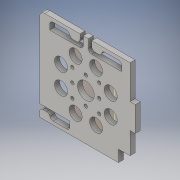
# Autodesk Inventor part: SideRotated
Saved by Autodesk Inventor 2016 SP1 (Build 200210100, 210)
## iProperties
Created: 2015-06-30
Part Number: SideRotated
Material: Generic
Document SubType Name: Modeling
Designer: Rodrigo
Density: 1 g/cm^3
Appearance: Default
Author: Rodrigo
Autodesk Inventor part; units mm, degrees
ref_plane "YZ Plane" through (0, 0, 0) normal (1, 0, 0) x (0, 1, 0)
ref_plane "XZ Plane" through (0, 0, 0) normal (0, 1, 0) x (-1, 0, 0)
ref_plane "XY Plane" through (0, 0, 0) normal (0, 0, 1) x (1, 0, 0)
ref_plane "Work Plane1" through (0, 0, 0) normal (0, 0, 1) x (1, 0, 0)
sketch "Sketch1" plane through (0, 0, 0) normal (0, 0, 1) x (1, 0, 0)
  circle A0 centre (6.5, 20.75) radius 1
  circle A1 centre (6.5, 4.75) radius 1
  circle A2 centre (22.5, 20.75) radius 1
  circle A3 centre (22.5, 4.75) radius 1
  line L0 (-13, -14.75) -> (43.896, -14.75)
  line L1 (43.896, -14.75) -> (43.896, 40.25)
  line L2 (43.896, 40.25) -> (-13, 40.25)
  line L3 (-13, 40.25) -> (-13, -14.75)
  circle A4 centre (22.5, 12.75) radius 1 projected
  circle A5 centre (14.5, 20.75) radius 1 projected
  circle A6 centre (14.5, 4.75) radius 1 projected
  circle A7 centre (6.5, 12.75) radius 1 projected
  point P0 (0, 0)
  point P1 (14.5, 12.75)
  dimension "d1" = 55
  dimension "d102" = 29.396
  dimension "d103" = 27.5
  dimension "d107" = 2
  dimension "d108" = 2
  dimension "d109" = 2
  dimension "d110" = 2
  constraints: 8 end point, 4 centre point, 2 parallel, 1 horizontal, 1 perpendicular
  measures "d1" distance of L1.end L0.end
  measures "d102" distance from line of L1 point (14.5, 12.75)
  measures "d103" distance from line of L3 point (14.5, 12.75)
  measures "d107" diameter of A0
  measures "d108" diameter of A2
  measures "d109" diameter of A3
  measures "d110" diameter of A1
extrude "Extrusion3" add sketch "Sketch1" along normal blind 3
sketch "Sketch4" plane through (0, 0, 3) normal (0, 0, 1) x (1, 0, 0)
  line L0 (42, 40.25) -> (-13, 40.25) construction
  line L1 (14.5, 40.25) -> (14.5, 12.75) construction
  line L2 (-13, 12.75) -> (14.5, 12.75) construction
  line L3 (42, 40.25) -> (-13, 40.25)
  line L4 (5, 38.2532) -> (-7, 38.25)
  line L5 (13, 40.25) -> (-7, 40.25)
  line L6 (-7, 38.25) -> (-7, 33.25)
  line L7 (-7, 33.25) -> (13, 33.25)
  line L8 (13, 40.25) -> (13, 33.25)
  line L9 (5, -7.75) -> (-13, -7.75)
  circle A0 centre (14.5, 12.75) radius 5
  line L10 (14.5, 12.75) -> (20.6229, 27.5321)
  line L11 (14.5, 12.75) -> (30.5, 12.75) construction
  circle A1 centre (20.6229, 27.5321) radius 3.895
  circle A2 centre (8.3771, 27.5321) radius 3.895
  circle A3 centre (-0.2821, 18.8729) radius 3.895
  circle A4 centre (-0.2821, 6.6271) radius 3.895
  circle A5 centre (8.3771, -2.0321) radius 3.895
  circle A6 centre (20.6229, -2.0321) radius 3.895
  circle A7 centre (29.2821, 6.6271) radius 3.895
  circle A8 centre (29.2821, 18.8729) radius 3.895
  line L12 (5, -12.75) -> (5, -7.75)
  line L13 (5, -12.75) -> (-7, -12.75)
  line L14 (-13, -7.75) -> (-13, -9.75)
  line L15 (-13, 40.25) -> (-13, -14.75) projected
  line L16 (-13, -9.75) -> (-7, -9.75)
  line L17 (-7, -9.75) -> (-7, -12.75)
  line L18 (-13, -14.75) -> (43.896, -14.75) projected
  line L19 (5, 38.2532) -> (5, 35.25)
  line L20 (5, 35.25) -> (11, 35.25)
  line L21 (11, 35.25) -> (11, 40.25)
  line L22 (24, 38.2532) -> (36, 38.25)
  line L23 (16, 40.25) -> (36, 40.25)
  line L24 (36, 38.25) -> (36, 33.25)
  line L25 (36, 33.25) -> (16, 33.25)
  line L26 (16, 40.25) -> (16, 33.25)
  line L27 (24, 38.2532) -> (24, 35.25)
  line L28 (24, 35.25) -> (18, 35.25)
  line L29 (18, 35.25) -> (18, 40.25)
  point P0 (0, 0)
  dimension "d66" = 20
  dimension "d105" = 10
  dimension "d111" = 16
  dimension "d112" = 67.5
  dimension "d113" = 7.79
  dimension "d116" = 360
  dimension "d119" = 12
  dimension "d120" = 2
  dimension "d121" = 5
  dimension "d122" = 2
  dimension "d123" = 18
  dimension "d124" = 2
  dimension "d125" = 5
  dimension "d126" = 2
  dimension "d127" = 2
  dimension "d128" = 6
  dimension "d129" = 12
  dimension "d130" = 6
  constraints: 56 end point, 9 centre point, 9 symmetric about line, 5 point on line, 4 horizontal, 4 perpendicular, 4 vertical, 2 coincident, 1 collinear, 1 equal length, 1 midpoint, 17 other
  measures "d66" distance of L5.start L5.end
  measures "d105" diameter of A0
  measures "d111" distance of L10.start L10.end
  measures "d112" angle of L11 L10
  measures "d113" diameter of A1
  measures "d119" distance of L12.start L13.end
  measures "d120" distance of L9.end L14.end
  measures "d121" distance between parallel lines of L18 L16
  measures "d122" distance between parallel lines of L18 L13
  measures "d123" distance of L9.start L9.end
  measures "d124" distance of L5.end L4.end
  measures "d125" distance of L20.end L21.end
  measures "d126" distance between parallel lines of L20 L7
  measures "d127" distance between parallel lines of L8 L21
  measures "d128" distance between parallel lines of L15 L6
  measures "d129" distance of L4.start L4.end
  measures "d130" distance of L19.end L20.end
extrude "Extrusion2" cut sketch "Sketch4" against normal through all
fillet "Fillet3" radius 2 14 edges at (-7, 38.25, 1.5) (5, 38.2532, 1.5) (13, 33.25, 1.5) (5, -12.75, 1.5) (-7, -12.75, 1.5) (-7, -9.75, 1.5) (-13, -9.75, 1.5) (5, 35.25, 1.5) (11, 35.25, 1.5) (16, 33.25, 1.5) (24, 35.25, 1.5) (18, 35.25, 1.5) (36, 38.25, 1.5) (24, 38.2532, 1.5)
sketch "Sketch6" plane through (0, 0, 3) normal (0, 0, 1) x (1, 0, 0)
  line L0 (43.896, 40.25) -> (-13, 40.25) projected
  line L1 (43.896, 40.25) -> (40.796, 40.25)
  line L2 (40.796, 40.25) -> (40.796, 20.2)
  line L3 (40.796, 20.2) -> (43.896, 20.2)
  line L4 (43.896, 20.2) -> (43.896, 40.25)
  line L5 (43.896, -14.75) -> (43.896, 40.25) construction
  line L6 (43.896, 12.75) -> (-13, 12.75) construction
  line L7 (-13, 40.25) -> (-13, -14.75) construction
  line L8 (43.896, -14.75) -> (40.796, -14.75)
  line L9 (40.796, -7.75) -> (40.796, 5.3)
  line L10 (40.796, 5.3) -> (43.896, 5.3)
  line L11 (43.896, 5.3) -> (43.896, -14.75)
  line L12 (43.896, -14.75) -> (33.896, -14.75)
  line L13 (33.896, -14.75) -> (33.896, -7.75)
  line L14 (33.896, -7.75) -> (40.796, -7.75)
  line L15 (43.896, -7.75) -> (43.896, -14.75)
  point P0 (0, 0)
  point P1 (36.3284, 40.25)
  point P2 (-13, -7.75)
  dimension "d96" = 3.1
  dimension "d97" = 20.05
  dimension "d100" = 10
  dimension "d101" = 7
  constraints: 26 end point, 4 parallel, 3 horizontal, 3 symmetric about line, 2 midpoint, 2 perpendicular
  measures "d96" distance of L3.end L2.end
  measures "d97" distance of L2.end L1.end
  measures "d100" distance of L13.end L15.start
  measures "d101" distance of L12.end L13.end
extrude "Extrusion4" cut sketch "Sketch6" against normal through all
fillet "Fillet4" radius 3 1 edges at (-13, 40.25, 1.5)
equation "\"d38\" = d24"
equation "\"d24\" = 7.79"
body "Solid1"
body "Solid2"
